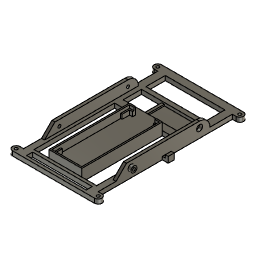
Car v2 (Autodesk Fusion 360 design; units mm, degrees)
Autodesk Fusion 360 part; units mm, degrees
note: some values were not read from the file. Set by a fixed rule: which sketch regions a step uses.
sketch "Structure" plane through (0, 0, 0) normal (0, 0, 1) x (1, 0, 0)
  line L0 (5, 0) -> (55, 0)
  line L1 (4.9996, 5) -> (5, 5)
  line L2 (5, 5) -> (5, 48)
  line L3 (4.9976, 100) -> (55, 100)
  arc A0 (55, 100) -> (54.9973, 100) centre (55, 97.5) ccw
  arc A1 (5.0024, 100) -> (4.9976, 100) centre (5, 97.5) ccw
  line L4 (10, 95) -> (10, 82)
  line L5 (10, 95) -> (50, 95)
  line L6 (50, 95) -> (50, 82)
  line L7 (10, 82) -> (50, 82)
  line L8 (10, 79) -> (10, 66.8)
  line L9 (23.6, 79) -> (10, 79)
  line L10 (10, 66.8) -> (23.6, 66.8)
  line L11 (23.6, 79) -> (23.6, 66.8)
  line L12 (4.9996, 8) -> (5, 8)
  line L13 (55, 5) -> (55, 8)
  line L14 (4.9996, 8) -> (5, 8)
  line L15 (10, 6) -> (50, 6)
  line L16 (10, 6) -> (10, 2)
  line L17 (10, 2) -> (50, 2)
  line L18 (50, 6) -> (50, 2)
  line L19 (19, 62) -> (19, 37)
  line L20 (19, 33) -> (19, 8)
  line L21 (19, 62) -> (9, 62)
  line L22 (19, 8) -> (9, 8)
  line L23 (9, 62) -> (9, 37)
  line L24 (9, 33) -> (9, 8)
  line L25 (41, 62) -> (41, 37)
  line L26 (41, 8) -> (41, 33)
  line L27 (41, 62) -> (51, 62)
  line L28 (41, 8) -> (51, 8)
  line L29 (51, 62) -> (51, 37)
  line L30 (51, 33) -> (51, 8)
  line L31 (55, 5) -> (55, 48)
  line L32 (55, 52) -> (59, 52)
  line L33 (55, 48) -> (59, 48)
  line L34 (59, 52) -> (59, 48)
  line L35 (55, 52) -> (55, 95)
  line L36 (5, 95) -> (5, 52)
  line L37 (5, 52) -> (1, 52)
  line L38 (1, 52) -> (1, 48)
  line L39 (1, 48) -> (5, 48)
  line L40 (9, 37) -> (9, 33)
  line L41 (19, 37) -> (19, 33)
  line L42 (41, 37) -> (41, 33)
  line L43 (51, 37) -> (51, 33)
  line L44 (55, 5) -> (57.5, 5)
  line L45 (55, 0) -> (57.5, 0)
  arc A2 (57.5, 0) -> (57.5, 5) centre (57.5, 2.5) ccw
  line L46 (55, 100) -> (57.5, 100)
  line L47 (55, 95) -> (57.5, 95)
  arc A3 (57.5, 95) -> (57.5, 100) centre (57.5, 97.5) ccw
  line L48 (5, 95) -> (2.5, 95)
  line L49 (5.0024, 100) -> (2.5024, 100)
  arc A4 (2.5024, 100) -> (2.5053, 95) centre (2.5, 97.5) ccw
  line L50 (4.9996, 5) -> (2.4996, 5)
  line L51 (5, 0) -> (2.5, 0)
  arc A5 (2.5006, 5) -> (2.5, 0) centre (2.5, 2.5) ccw
  dimension "d4" = 90
  dimension "d7" = 90
  dimension "d13" = 5
  dimension "d14" = 5
  dimension "d17" = 5
  dimension "d18" = 13
  dimension "d19" = 40
  dimension "d20" = 13
  dimension "d21" = 40
  dimension "d22" = 3
  dimension "d23" = 12.2
  dimension "d28" = 13.6
  dimension "d29" = 13.6
  dimension "d30" = 12.2
  dimension "d31" = 3
  dimension "d33" = 3
  dimension "d42" = 54
  dimension "d43" = 54
  dimension "d47" = 40
  dimension "d48" = 4
  dimension "d49" = 40
  dimension "d50" = 4
  dimension "d51" = 25
  dimension "d53" = 4
  dimension "d55" = 10
  dimension "d57" = 10
  dimension "d58" = 10
  dimension "d59" = 25
  dimension "d60" = 25
  dimension "d61" = 25
  dimension "d62" = 25
  dimension "d63" = 10
  dimension "d65" = 10
  dimension "d66" = 10
  dimension "d67" = 25
  dimension "d68" = 25
  dimension "d82" = 43
  dimension "d83" = 43
  dimension "d84" = 4
  dimension "d85" = 4
  dimension "d86" = 43
  dimension "d87" = 4
  dimension "d88" = 4
  dimension "d89" = 4
  dimension "d239" = 2.5
  dimension "d240" = 2.5
  dimension "d241" = 2.5
  dimension "d242" = 2.5
  dimension "d243" = 5
  dimension "d244" = 2.5
  dimension "d245" = 2.5
  dimension "d246" = 2.5
  dimension "d247" = 2.5
  constraint horizontal L0
  constraint perpendicular L1 L2
  constraint coincident L3 A0.end
  constraint coincident L3 A1.start
  constraint perpendicular L5 L6
  constraint perpendicular L6 L7
  constraint perpendicular L8 L9
  constraint perpendicular L8 L10
  constraint perpendicular L10 L11
  constraint perpendicular L2 L14
  constraint coincident L2 L12.end
  constraint perpendicular L15 L16
  constraint perpendicular L16 L17
  constraint perpendicular L15 L18
  constraint perpendicular L19 L21
  constraint perpendicular L20 L22
  constraint perpendicular L21 L23
  constraint perpendicular L25 L27
  constraint perpendicular L26 L28
  constraint perpendicular L27 L29
  constraint perpendicular L31 L33
  constraint parallel L2 L36
  constraint perpendicular L36 L37
  constraint perpendicular L37 L38
  constraint perpendicular L38 L39
  constraint parallel L24 L40
  constraint parallel L20 L41
  constraint parallel L26 L42
  constraint parallel L30 L43
  constraint perpendicular L31 L44
  constraint parallel L0 L45
  constraint parallel L3 L46
  constraint perpendicular L35 L47
  constraint perpendicular L36 L48
  constraint parallel L3 L49
  constraint coincident L48 A4.end
  constraint perpendicular L2 L50
  constraint parallel L0 L51
  constraint coincident L50 A5.start
  measures "d4" distance of L13.start L35.end
  measures "d7" distance of L1.end L36.start
  measures "d13" diameter of A0
  measures "d14" diameter of A1
  measures "d17" distance of L36.start L4.start
  measures "d18" distance of L4.start L4.end
  measures "d19" distance of L4.start L5.end
  measures "d20" distance of L5.end L6.end
  measures "d21" distance of L4.end L6.end
  measures "d22" distance of L4.end L8.start
  measures "d23" distance of L8.start L8.end
  measures "d28" distance of L9.start L8.start
  measures "d29" distance of L8.end L10.end
  measures "d30" distance of L9.start L10.end
  measures "d31" distance of L1.start L12.start
  measures "d33" distance of L13.start L13.end
  measures "d42" distance of L19.start L20.end
  measures "d43" distance of L26.start L25.start
  measures "d47" distance of L15.start L15.end
  measures "d48" distance of L15.start L16.end
  measures "d49" distance of L16.end L17.end
  measures "d50" distance of L15.end L17.end
  measures "d51" distance of L19.start L19.end
  measures "d53" distance of L19.end L20.start
  measures "d55" distance of L19.start L21.end
  measures "d57" distance of L20.start L24.start
  measures "d58" distance of L20.end L22.end
  measures "d59" distance of L21.end L23.end
  measures "d60" distance of L24.start L22.end
  measures "d61" distance of L25.start L25.end
  measures "d62" distance of L26.start L26.end
  measures "d63" distance of L25.start L27.end
  measures "d65" distance of L26.end L30.start
  measures "d66" distance of L26.start L28.end
  measures "d67" distance of L27.end L29.end
  measures "d68" distance of L30.start L28.end
  measures "d82" distance of L35.end L32.start
  measures "d83" distance of L13.start L31.end
  measures "d84" distance of L32.start L32.end
  measures "d85" distance of L31.end L33.end
  measures "d86" distance of L36.start L36.end
  measures "d87" distance of L36.end L37.end
  measures "d88" distance of L37.end L38.end
  measures "d89" distance of L38.end L2.end
  measures "d239" distance of L13.start L44.end
  measures "d240" distance of L0.end L45.end
  measures "d241" distance of L3.end L46.end
  measures "d242" distance of L35.end L47.end
  measures "d243" diameter of A3
  measures "d244" distance of L36.start L48.end
  measures "d245" distance of A1.start L49.end
  measures "d246" distance of L1.start L50.end
  measures "d247" distance of L0.start L51.end
extrude "Extrude1" add sketch "Structure" along normal blind 3
sketch "Motor Hole" plane through (0, 0, 3) normal (0, 0, 1) x (-1, 0, 0)
  line L0 (-10, -82) -> (-10, -95)
  line L1 (-10, -95) -> (-50, -95)
  line L2 (-50, -95) -> (-50, -82)
  line L3 (-50, -82) -> (-10, -82)
  line L4 (-9, -62) -> (-19, -62)
  line L5 (-19, -62) -> (-19, -8)
  line L6 (-9, -8) -> (-9, -62)
  line L7 (-10, -2) -> (-10, -6)
  line L8 (-10, -6) -> (-50, -6)
  line L9 (-50, -6) -> (-50, -2)
  line L10 (-50, -2) -> (-10, -2)
  line L11 (-10, -66.8) -> (-10, -79)
  line L12 (-10, -79) -> (-23.6, -79)
  line L13 (-23.6, -79) -> (-23.6, -66.8)
  line L14 (-23.6, -66.8) -> (-10, -66.8)
  line L15 (-41, -8) -> (-41, -62)
  line L16 (-41, -62) -> (-51, -62)
  line L17 (-51, -62) -> (-51, -8)
  line L18 (-19, -8) -> (-9, -8)
  line L19 (-51, -8) -> (-41, -8)
  line L20 (-2.5, 0) -> (-57.5, 0)
  line L21 (-55, -5) -> (-55, -48)
  arc A0 (-55, -100) -> (-54.9973, -100) centre (-55, -97.5) ccw
  line L22 (-5, -48) -> (-5, -5)
  line L23 (-50, -79) -> (-50, -66.8)
  line L24 (-50, -79) -> (-25.6, -79)
  line L25 (-25.6, -79) -> (-25.6, -66.8)
  line L26 (-25.6, -66.8) -> (-50, -66.8)
  line L27 (-23.6, -79) -> (-25.6, -79)
  line L28 (-23.6, -66.8) -> (-25.6, -66.8)
  line L29 (-5, -95) -> (-5, -52)
  line L30 (-5, -52) -> (-1, -52)
  line L31 (-1, -52) -> (-1, -48)
  line L32 (-1, -48) -> (-5, -48)
  line L33 (-55, -48) -> (-59, -48)
  line L34 (-59, -48) -> (-59, -52)
  line L35 (-59, -52) -> (-55, -52)
  line L36 (-55, -52) -> (-55, -95)
  line L37 (-5, -5) -> (-2.5006, -5)
  arc A1 (-2.5006, -5) -> (-2.5, 0) centre (-2.5, -2.5) ccw
  arc A2 (-57.5, 0) -> (-57.5, -5) centre (-57.5, -2.5) ccw
  line L38 (-57.5, -5) -> (-55, -5)
  line L39 (-55, -95) -> (-57.5, -95)
  arc A3 (-57.5, -95) -> (-57.5, -100) centre (-57.5, -97.5) ccw
  line L40 (-57.5, -100) -> (-55, -100)
  line L41 (-54.9973, -100) -> (-2.5024, -100)
  arc A4 (-2.5024, -100) -> (-2.5053, -95) centre (-2.5, -97.5) ccw
  line L42 (-2.5053, -95) -> (-5, -95)
  dimension "d71" = 3
  dimension "d72" = 12.2
  dimension "d73" = 24.4
  dimension "d74" = 12.2
  dimension "d75" = 24.4
  dimension "d76" = 2
  dimension "d77" = 2
  constraint perpendicular L3 L23
  constraint perpendicular L23 L24
  constraint perpendicular L24 L25
  constraint perpendicular L25 L26
  constraint coincident L12.end L13.start
  constraint perpendicular L25 L27
  constraint coincident L13.end L14.start
  constraint perpendicular L25 L28
  measures "d71" distance of L2.end L23.start
  measures "d72" distance of L23.start L23.end
  measures "d73" distance of L23.start L24.end
  measures "d74" distance of L24.end L25.end
  measures "d75" distance of L25.end L23.end
  measures "d76" distance of L12.end L24.end
  measures "d77" distance of L13.end L25.end
extrude "Extrude2" cut sketch "Motor Hole" against normal blind 2 contours L23 L24 L25 L26
extrude "Extrude3" cut sketch "Motor Hole" against normal blind 1 contours L13 L25 L27 L28
sketch "Rec. Base1" plane through (0, 0, 3) normal (0, 0, 1) x (-1, 0, 0)
  line L0 (-2.5, 0) -> (-57.5, 0)
  line L1 (-55, -5) -> (-55, -48)
  arc A0 (-55, -100) -> (-54.9973, -100) centre (-55, -97.5) ccw
  line L2 (-5, -48) -> (-5, -5)
  line L3 (-51, -8) -> (-41, -8)
  line L4 (-19, -8) -> (-9, -8)
  line L5 (-41, -8) -> (-41, -62)
  line L6 (-41, -62) -> (-51, -62)
  line L7 (-51, -62) -> (-51, -8)
  line L8 (-50, -66.8) -> (-10, -66.8)
  line L9 (-10, -66.8) -> (-10, -79)
  line L10 (-10, -79) -> (-50, -79)
  line L11 (-50, -79) -> (-50, -66.8)
  line L12 (-10, -2) -> (-10, -6)
  line L13 (-10, -6) -> (-50, -6)
  line L14 (-50, -6) -> (-50, -2)
  line L15 (-50, -2) -> (-10, -2)
  line L16 (-9, -62) -> (-19, -62)
  line L17 (-19, -62) -> (-19, -8)
  line L18 (-9, -8) -> (-9, -62)
  line L19 (-10, -82) -> (-10, -95)
  line L20 (-10, -95) -> (-50, -95)
  line L21 (-50, -95) -> (-50, -82)
  line L22 (-50, -82) -> (-10, -82)
  line L23 (-5, -95) -> (-5, -52)
  line L24 (-5, -52) -> (-1, -52)
  line L25 (-1, -52) -> (-1, -48)
  line L26 (-1, -48) -> (-5, -48)
  line L27 (-55, -48) -> (-59, -48)
  line L28 (-59, -48) -> (-59, -52)
  line L29 (-59, -52) -> (-55, -52)
  line L30 (-55, -52) -> (-55, -95)
  line L31 (-19, -8) -> (-41, -8)
  line L32 (-19, -8) -> (-19, -62)
  line L33 (-41, -8) -> (-41, -62)
  line L34 (-19, -62) -> (-26, -62)
  line L35 (-41, -62) -> (-34, -62)
  line L36 (-26, -62) -> (-26, -61)
  line L37 (-34, -62) -> (-34, -61)
  line L38 (-26, -61) -> (-20, -61)
  line L39 (-34, -61) -> (-40, -61)
  line L40 (-20, -61) -> (-20, -9)
  line L41 (-20, -9) -> (-40, -9)
  line L42 (-40, -9) -> (-40, -61)
  line L43 (-5, -5) -> (-2.5006, -5)
  arc A1 (-2.5006, -5) -> (-2.5, 0) centre (-2.5, -2.5) ccw
  arc A2 (-57.5, 0) -> (-57.5, -5) centre (-57.5, -2.5) ccw
  line L44 (-57.5, -5) -> (-55, -5)
  line L45 (-55, -95) -> (-57.5, -95)
  arc A3 (-57.5, -95) -> (-57.5, -100) centre (-57.5, -97.5) ccw
  line L46 (-57.5, -100) -> (-55, -100)
  line L47 (-54.9973, -100) -> (-2.5024, -100)
  arc A4 (-2.5024, -100) -> (-2.5053, -95) centre (-2.5, -97.5) ccw
  line L48 (-2.5053, -95) -> (-5, -95)
  dimension "d90" = 22
  dimension "d91" = 54
  dimension "d92" = 54
  dimension "d93" = 7
  dimension "d94" = 7
  dimension "d95" = 1
  dimension "d96" = 1
  dimension "d97" = 6
  dimension "d98" = 6
  dimension "d99" = 52
  dimension "d100" = 20
  dimension "d101" = 52
  constraint coincident L4.start L17.end
  constraint perpendicular L16 L32
  constraint perpendicular L6 L33
  constraint coincident L16.end L17.start
  constraint perpendicular L32 L34
  constraint coincident L5.end L6.start
  constraint perpendicular L33 L35
  constraint perpendicular L34 L36
  constraint perpendicular L35 L37
  constraint perpendicular L36 L38
  constraint perpendicular L37 L39
  constraint perpendicular L38 L40
  constraint perpendicular L32 L41
  constraint perpendicular L41 L42
  measures "d90" distance of L4.start L3.end
  measures "d91" distance of L4.start L16.end
  measures "d92" distance of L3.end L5.end
  measures "d93" distance of L16.end L34.end
  measures "d94" distance of L5.end L35.end
  measures "d95" distance of L34.end L36.end
  measures "d96" distance of L35.end L37.end
  measures "d97" distance of L36.end L38.end
  measures "d98" distance of L37.end L39.end
  measures "d99" distance of L38.end L40.end
  measures "d100" distance of L40.end L41.end
  measures "d101" distance of L41.end L39.end
extrude "Extrude4" add sketch "Rec. Base1" along normal blind 7 contours L5 L17 L31 L32 L33 L34 L35 L36 L37 L38 L39 L40 L41 L42
sketch "Hook" plane through (0, 0, 3) normal (0, 0, 1) x (-1, 0, 0)
  line L0 (-34, -62) -> (-41, -62)
  line L1 (-41, -62) -> (-51, -62)
  line L2 (-51, -62) -> (-51, -8)
  line L3 (-51, -8) -> (-41, -8)
  line L4 (-41, -8) -> (-19, -8)
  line L5 (-19, -8) -> (-9, -8)
  line L6 (-9, -8) -> (-9, -62)
  line L7 (-9, -62) -> (-19, -62)
  line L8 (-19, -62) -> (-26, -62)
  line L9 (-26, -62) -> (-26, -61)
  line L10 (-26, -61) -> (-20, -61)
  line L11 (-20, -61) -> (-20, -9)
  line L12 (-20, -9) -> (-40, -9)
  line L13 (-40, -9) -> (-40, -61)
  line L14 (-40, -61) -> (-34, -61)
  line L15 (-34, -61) -> (-34, -62)
  arc A0 (-55, -100) -> (-54.9973, -100) centre (-55, -97.5) ccw
  line L16 (-5, -95) -> (-5, -52)
  line L17 (-5, -52) -> (-1, -52)
  line L18 (-1, -52) -> (-1, -48)
  line L19 (-1, -48) -> (-5, -48)
  line L20 (-5, -48) -> (-5, -5)
  line L21 (-2.5, 0) -> (-57.5, 0)
  line L22 (-55, -5) -> (-55, -48)
  line L23 (-55, -48) -> (-59, -48)
  line L24 (-59, -48) -> (-59, -52)
  line L25 (-59, -52) -> (-55, -52)
  line L26 (-55, -52) -> (-55, -95)
  line L27 (-10, -2) -> (-10, -6)
  line L28 (-10, -6) -> (-50, -6)
  line L29 (-50, -6) -> (-50, -2)
  line L30 (-50, -2) -> (-10, -2)
  line L31 (-50, -66.8) -> (-10, -66.8)
  line L32 (-10, -66.8) -> (-10, -79)
  line L33 (-10, -79) -> (-50, -79)
  line L34 (-50, -79) -> (-50, -66.8)
  line L35 (-10, -82) -> (-10, -95)
  line L36 (-10, -95) -> (-50, -95)
  line L37 (-50, -95) -> (-50, -82)
  line L38 (-50, -82) -> (-10, -82)
  line L39 (-57, -52) -> (-57, -48)
  line L40 (-55, -52) -> (-55, -48)
  line L41 (-5, -52) -> (-5, -48)
  line L42 (-3, -52) -> (-3, -48)
  line L43 (-5, -5) -> (-2.5006, -5)
  arc A1 (-2.5006, -5) -> (-2.5, 0) centre (-2.5, -2.5) ccw
  arc A2 (-57.5, 0) -> (-57.5, -5) centre (-57.5, -2.5) ccw
  line L44 (-57.5, -5) -> (-55, -5)
  line L45 (-55, -95) -> (-57.5, -95)
  arc A3 (-57.5, -95) -> (-57.5, -100) centre (-57.5, -97.5) ccw
  line L46 (-57.5, -100) -> (-55, -100)
  line L47 (-54.9973, -100) -> (-2.5024, -100)
  arc A4 (-2.5024, -100) -> (-2.5053, -95) centre (-2.5, -97.5) ccw
  line L48 (-2.5053, -95) -> (-5, -95)
  constraint midpoint L25 L39.start
  constraint midpoint L23 L39.end
  constraint coincident L25.end L26.start
  constraint coincident L22.end L23.start
  constraint coincident L16.end L17.start
  constraint coincident L19.end L20.start
  constraint midpoint L17 L42.start
  constraint midpoint L19 L42.end
extrude "Extrude5" cut sketch "Hook" against normal blind 1 contours L23 L25 L39 L40
extrude "Extrude6" add 1 faces at (57.6667, 50.6667, 3) along direction (0, 0, 1) blind 1
extrude "Extrude7" cut sketch "Hook" against normal blind 1 contours L17 L19 L41 L42
extrude "Extrude8" add sketch "Hook" along normal blind 1 contours L17 L18 L19 L42
sketch "Rec. Base2" plane through (0, 0, 3) normal (0, 0, 1) x (-1, 0, 0)
  line L0 (-5, -95) -> (-5, -5)
  line L1 (-2.5, 0) -> (-57.5, 0)
  line L2 (-55, -5) -> (-55, -95)
  arc A0 (-55, -100) -> (-54.9973, -100) centre (-55, -97.5) ccw
  line L3 (-34, -62) -> (-41, -62)
  line L4 (-41, -62) -> (-51, -62)
  line L5 (-51, -62) -> (-51, -8)
  line L6 (-51, -8) -> (-41, -8)
  line L7 (-41, -8) -> (-19, -8)
  line L8 (-19, -8) -> (-9, -8)
  line L9 (-9, -8) -> (-9, -62)
  line L10 (-9, -62) -> (-19, -62)
  line L11 (-19, -62) -> (-26, -62)
  line L12 (-26, -62) -> (-26, -61)
  line L13 (-26, -61) -> (-20, -61)
  line L14 (-20, -61) -> (-20, -9)
  line L15 (-20, -9) -> (-40, -9)
  line L16 (-40, -9) -> (-40, -61)
  line L17 (-40, -61) -> (-34, -61)
  line L18 (-34, -61) -> (-34, -62)
  line L19 (-10, -2) -> (-10, -6)
  line L20 (-10, -6) -> (-50, -6)
  line L21 (-50, -6) -> (-50, -2)
  line L22 (-50, -2) -> (-10, -2)
  line L23 (-50, -66.8) -> (-10, -66.8)
  line L24 (-10, -66.8) -> (-10, -79)
  line L25 (-10, -79) -> (-50, -79)
  line L26 (-50, -79) -> (-50, -66.8)
  line L27 (-10, -82) -> (-10, -95)
  line L28 (-10, -95) -> (-50, -95)
  line L29 (-50, -95) -> (-50, -82)
  line L30 (-50, -82) -> (-10, -82)
  line L31 (-20, -58) -> (-21, -58)
  line L32 (-21, -58) -> (-21, -60)
  line L33 (-21, -60) -> (-23, -60)
  line L34 (-23, -60) -> (-23, -61)
  line L35 (-40, -58) -> (-39, -58)
  line L36 (-39, -58) -> (-39, -60)
  line L37 (-39, -60) -> (-37, -60)
  line L38 (-37, -60) -> (-37, -61)
  line L39 (-20, -12) -> (-21, -12)
  line L40 (-21, -12) -> (-21, -10)
  line L41 (-21, -10) -> (-23, -10)
  line L42 (-23, -10) -> (-23, -9)
  line L43 (-40, -12) -> (-39, -12)
  line L44 (-39, -12) -> (-39, -10)
  line L45 (-39, -10) -> (-37, -10)
  line L46 (-37, -10) -> (-37, -9)
  line L47 (-5, -5) -> (-2.5006, -5)
  arc A1 (-2.5006, -5) -> (-2.5, 0) centre (-2.5, -2.5) ccw
  arc A2 (-57.5, 0) -> (-57.5, -5) centre (-57.5, -2.5) ccw
  line L48 (-57.5, -5) -> (-55, -5)
  line L49 (-55, -95) -> (-57.5, -95)
  arc A3 (-57.5, -95) -> (-57.5, -100) centre (-57.5, -97.5) ccw
  line L50 (-57.5, -100) -> (-55, -100)
  line L51 (-54.9973, -100) -> (-2.5024, -100)
  arc A4 (-2.5024, -100) -> (-2.5053, -95) centre (-2.5, -97.5) ccw
  line L52 (-2.5053, -95) -> (-5, -95)
  dimension "d112" = 3
  dimension "d113" = 1
  dimension "d114" = 2
  dimension "d115" = 2
  dimension "d116" = 1
  dimension "d117" = 3
  dimension "d118" = 1
  dimension "d119" = 2
  dimension "d120" = 2
  dimension "d121" = 1
  dimension "d122" = 3
  dimension "d123" = 1
  dimension "d124" = 2
  dimension "d125" = 2
  dimension "d126" = 1
  dimension "d127" = 3
  dimension "d128" = 1
  dimension "d129" = 2
  dimension "d130" = 2
  dimension "d131" = 1
  constraint perpendicular L31 L32
  constraint perpendicular L32 L33
  constraint perpendicular L13 L34
  constraint perpendicular L35 L36
  constraint perpendicular L36 L37
  constraint perpendicular L37 L38
  constraint perpendicular L39 L40
  constraint perpendicular L40 L41
  constraint perpendicular L41 L42
  constraint perpendicular L43 L44
  constraint perpendicular L44 L45
  constraint perpendicular L45 L46
  measures "d112" distance of L13.end L31.start
  measures "d113" distance of L31.start L31.end
  measures "d114" distance of L31.end L32.end
  measures "d115" distance of L32.end L33.end
  measures "d116" distance of L33.end L34.end
  measures "d117" distance of L16.end L35.start
  measures "d118" distance of L35.start L35.end
  measures "d119" distance of L35.end L36.end
  measures "d120" distance of L36.end L37.end
  measures "d121" distance of L37.end L38.end
  measures "d122" distance of L14.end L39.start
  measures "d123" distance of L39.start L39.end
  measures "d124" distance of L39.end L40.end
  measures "d125" distance of L40.end L41.end
  measures "d126" distance of L41.end L42.end
  measures "d127" distance of L15.end L43.start
  measures "d128" distance of L43.start L43.end
  measures "d129" distance of L43.end L44.end
  measures "d130" distance of L44.end L45.end
  measures "d131" distance of L45.end L46.end
extrude "Extrude9" cut 1 faces at (40.6667, 26.3333, 10) along direction (0, 0, -1) blind 2
extrude "Extrude10" add sketch "Rec. Base2" along normal blind 3 contours L13 L14 L31 L32 L33 L34
extrude "Extrude11" add sketch "Rec. Base2" along normal blind 3 contours L16 L17 L35 L36 L37 L38
extrude "Extrude12" add sketch "Rec. Base2" along normal blind 3 contours L15 L16 L43 L44 L45 L46
extrude "Extrude13" add sketch "Rec. Base2" along normal blind 3 contours L14 L15 L39 L40 L41 L42
sketch "Side Wheel Base" plane through (0, 0, 3) normal (0, 0, 1) x (-1, 0, 0)
  line L0 (-5, -95) -> (-5, -5)
  line L1 (-2.5, 0) -> (-57.5, 0)
  line L2 (-55, -5) -> (-55, -95)
  arc A0 (-55, -100) -> (-54.9973, -100) centre (-55, -97.5) ccw
  line L3 (-10, -2) -> (-10, -6)
  line L4 (-10, -6) -> (-50, -6)
  line L5 (-50, -6) -> (-50, -2)
  line L6 (-50, -2) -> (-10, -2)
  line L7 (-50, -66.8) -> (-10, -66.8)
  line L8 (-10, -66.8) -> (-10, -79)
  line L9 (-10, -79) -> (-50, -79)
  line L10 (-50, -79) -> (-50, -66.8)
  line L11 (-10, -82) -> (-10, -95)
  line L12 (-10, -95) -> (-50, -95)
  line L13 (-50, -95) -> (-50, -82)
  line L14 (-50, -82) -> (-10, -82)
  line L15 (-20, -12) -> (-21, -12)
  line L16 (-21, -12) -> (-21, -10)
  line L17 (-21, -10) -> (-23, -10)
  line L18 (-23, -10) -> (-23, -9)
  line L19 (-23, -9) -> (-37, -9)
  line L20 (-37, -9) -> (-37, -10)
  line L21 (-37, -10) -> (-39, -10)
  line L22 (-39, -10) -> (-39, -12)
  line L23 (-39, -12) -> (-40, -12)
  line L24 (-40, -12) -> (-40, -58)
  line L25 (-40, -58) -> (-39, -58)
  line L26 (-39, -58) -> (-39, -60)
  line L27 (-39, -60) -> (-37, -60)
  line L28 (-37, -60) -> (-37, -61)
  line L29 (-37, -61) -> (-34, -61)
  line L30 (-34, -61) -> (-34, -62)
  line L31 (-34, -62) -> (-41, -62)
  line L32 (-41, -62) -> (-51, -62)
  line L33 (-51, -62) -> (-51, -8)
  line L34 (-51, -8) -> (-41, -8)
  line L35 (-41, -8) -> (-19, -8)
  line L36 (-19, -8) -> (-9, -8)
  line L37 (-9, -8) -> (-9, -62)
  line L38 (-9, -62) -> (-19, -62)
  line L39 (-19, -62) -> (-26, -62)
  line L40 (-26, -62) -> (-26, -61)
  line L41 (-26, -61) -> (-23, -61)
  line L42 (-23, -61) -> (-23, -60)
  line L43 (-23, -60) -> (-21, -60)
  line L44 (-21, -60) -> (-21, -58)
  line L45 (-21, -58) -> (-20, -58)
  line L46 (-20, -58) -> (-20, -12)
  circle A1 centre (-5, -2.5) radius 1.5
  circle A2 centre (-55, -2.5) radius 1.5
  circle A3 centre (-55, -97.5) radius 1.5
  circle A4 centre (-5, -97.5) radius 1.5
  circle A5 centre (-5, -97.5) radius 0.9
  circle A6 centre (-55, -97.5) radius 0.9
  circle A7 centre (-55, -2.5) radius 0.9
  circle A8 centre (-5, -2.5) radius 0.9
  line L47 (-5, -5) -> (-2.5006, -5)
  arc A9 (-2.5006, -5) -> (-2.5, 0) centre (-2.5, -2.5) ccw
  arc A10 (-57.5, 0) -> (-57.5, -5) centre (-57.5, -2.5) ccw
  line L48 (-57.5, -5) -> (-55, -5)
  line L49 (-55, -95) -> (-57.5, -95)
  arc A11 (-57.5, -95) -> (-57.5, -100) centre (-57.5, -97.5) ccw
  line L50 (-57.5, -100) -> (-55, -100)
  line L51 (-54.9973, -100) -> (-2.5024, -100)
  arc A12 (-2.5024, -100) -> (-2.5053, -95) centre (-2.5, -97.5) ccw
  line L52 (-2.5053, -95) -> (-5, -95)
  dimension "d142" = 3
  dimension "d143" = 3
  dimension "d144" = 3
  dimension "d145" = 3
  dimension "d146" = 1.8
  dimension "d147" = 1.8
  dimension "d148" = 1.8
  dimension "d149" = 1.8
  constraint concentric A0 A3
  constraint concentric A4 A5
  constraint concentric A3 A6
  constraint concentric A2 A7
  constraint concentric A1 A8
  measures "d142" diameter of A1
  measures "d143" diameter of A2
  measures "d144" diameter of A3
  measures "d145" diameter of A4
  measures "d146" diameter of A5
  measures "d147" diameter of A6
  measures "d148" diameter of A7
  measures "d149" diameter of A8
extrude "Extrude14" add sketch "Side Wheel Base" along normal blind 3.4 contours A8
extrude "Extrude15" add sketch "Side Wheel Base" along normal blind 1 contours A1
extrude "Extrude16" add sketch "Side Wheel Base" along normal blind 3.4 contours A7
extrude "Extrude17" add sketch "Side Wheel Base" along normal blind 1 contours A2
extrude "Extrude18" add sketch "Side Wheel Base" along normal blind 3.4 contours A6
extrude "Extrude19" add sketch "Side Wheel Base" along normal blind 1 contours A3
extrude "Extrude20" add sketch "Side Wheel Base" along normal blind 3.4 contours A5
extrude "Extrude21" add sketch "Side Wheel Base" along normal blind 1 contours A4
sketch "Side Car1" plane through (0, 0, 3) normal (0, 0, 1) x (-1, 0, 0)
  circle A0 centre (-5, -97.5) radius 1.5
  circle A1 centre (-55, -97.5) radius 1.5
  circle A2 centre (-55, -2.5) radius 1.5
  circle A3 centre (-5, -2.5) radius 1.5
  line L0 (-5, -95) -> (-5, -5)
  line L1 (-2.5, 0) -> (-57.5, 0)
  line L2 (-55, -5) -> (-55, -95)
  arc A4 (-55, -100) -> (-54.9973, -100) centre (-55, -97.5) ccw
  line L3 (-10, -2) -> (-10, -6)
  line L4 (-10, -6) -> (-50, -6)
  line L5 (-50, -6) -> (-50, -2)
  line L6 (-50, -2) -> (-10, -2)
  line L7 (-50, -66.8) -> (-10, -66.8)
  line L8 (-10, -66.8) -> (-10, -79)
  line L9 (-10, -79) -> (-50, -79)
  line L10 (-50, -79) -> (-50, -66.8)
  line L11 (-10, -82) -> (-10, -95)
  line L12 (-10, -95) -> (-50, -95)
  line L13 (-50, -95) -> (-50, -82)
  line L14 (-50, -82) -> (-10, -82)
  line L15 (-20, -12) -> (-21, -12)
  line L16 (-21, -12) -> (-21, -10)
  line L17 (-21, -10) -> (-23, -10)
  line L18 (-23, -10) -> (-23, -9)
  line L19 (-23, -9) -> (-37, -9)
  line L20 (-37, -9) -> (-37, -10)
  line L21 (-37, -10) -> (-39, -10)
  line L22 (-39, -10) -> (-39, -12)
  line L23 (-39, -12) -> (-40, -12)
  line L24 (-40, -12) -> (-40, -58)
  line L25 (-40, -58) -> (-39, -58)
  line L26 (-39, -58) -> (-39, -60)
  line L27 (-39, -60) -> (-37, -60)
  line L28 (-37, -60) -> (-37, -61)
  line L29 (-37, -61) -> (-34, -61)
  line L30 (-34, -61) -> (-34, -62)
  line L31 (-34, -62) -> (-41, -62)
  line L32 (-41, -62) -> (-51, -62)
  line L33 (-51, -62) -> (-51, -8)
  line L34 (-51, -8) -> (-41, -8)
  line L35 (-41, -8) -> (-19, -8)
  line L36 (-19, -8) -> (-9, -8)
  line L37 (-9, -8) -> (-9, -62)
  line L38 (-9, -62) -> (-19, -62)
  line L39 (-19, -62) -> (-26, -62)
  line L40 (-26, -62) -> (-26, -61)
  line L41 (-26, -61) -> (-23, -61)
  line L42 (-23, -61) -> (-23, -60)
  line L43 (-23, -60) -> (-21, -60)
  line L44 (-21, -60) -> (-21, -58)
  line L45 (-21, -58) -> (-20, -58)
  line L46 (-20, -58) -> (-20, -12)
  line L47 (-55, -80) -> (-53, -80)
  line L48 (-55, -17) -> (-53, -17)
  line L49 (-53, -80) -> (-53, -17)
  line L50 (-5, -80) -> (-7, -80)
  line L51 (-7, -80) -> (-7, -17)
  line L52 (-5, -17) -> (-7, -17)
  line L53 (-5, -5) -> (-2.5006, -5)
  arc A5 (-2.5006, -5) -> (-2.5, 0) centre (-2.5, -2.5) ccw
  arc A6 (-57.5, 0) -> (-57.5, -5) centre (-57.5, -2.5) ccw
  line L54 (-57.5, -5) -> (-55, -5)
  line L55 (-55, -95) -> (-57.5, -95)
  arc A7 (-57.5, -95) -> (-57.5, -100) centre (-57.5, -97.5) ccw
  line L56 (-57.5, -100) -> (-55, -100)
  line L57 (-54.9973, -100) -> (-2.5024, -100)
  arc A8 (-2.5024, -100) -> (-2.5053, -95) centre (-2.5, -97.5) ccw
  line L58 (-2.5053, -95) -> (-5, -95)
  dimension "d166" = 12
  dimension "d167" = 15
  dimension "d168" = 2
  dimension "d169" = 2
  dimension "d170" = 63
  dimension "d171" = 15
  dimension "d172" = 12
  dimension "d173" = 2
  dimension "d174" = 63
  dimension "d175" = 2
  constraint perpendicular L48 L49
  constraint perpendicular L50 L51
  constraint perpendicular L51 L52
  measures "d166" distance of L2.start L48.start
  measures "d167" distance of L2.end L47.start
  measures "d168" distance of L47.start L47.end
  measures "d169" distance of L48.start L48.end
  measures "d170" distance of L47.end L48.end
  measures "d171" distance of L0.start L50.start
  measures "d172" distance of L0.end L52.start
  measures "d173" distance of L50.start L50.end
  measures "d174" distance of L50.end L51.end
  measures "d175" distance of L52.start L51.end
extrude "Extrude22" add sketch "Side Car1" along normal blind 7 contours L0 L50 L51 L52
extrude "Extrude23" add sketch "Side Car1" along normal blind 7 contours L2 L47 L48 L49
sketch "Left Side Car" plane through (55, 0, 0) normal (1, 0, 0) x (0, 1, 0)
  line L0 (52, 0) -> (95, 0)
  line L1 (95, 3) -> (80, 3)
  line L2 (80, 3) -> (80, 10)
  line L3 (80, 10) -> (17, 10)
  line L4 (17, 10) -> (17, 3)
  line L5 (48, 0) -> (48, 2)
  line L6 (48, 2) -> (52, 2)
  line L7 (52, 2) -> (52, 0)
  line L8 (17, 3) -> (24, 10)
  arc A0 (80, 3) -> (73, 10) centre (73, 3) ccw
  line L9 (95, 0) -> (95, 3)
  line L10 (17, 3) -> (5, 3)
  line L11 (5, 3) -> (5, 0)
  line L12 (5, 0) -> (48, 0)
  dimension "d182" = 7
  dimension "d183" = 14
  constraint coincident L4.end L8.start
  constraint coincident L3 A0.end
  measures "d182" distance of L1.end A0.centre
  measures "d183" diameter of A0
extrude "Extrude24" cut sketch "Left Side Car" against normal blind 3 contours L3 L4 L8
extrude "Extrude25" cut sketch "Left Side Car" against normal blind 3 contours L2 L3 A0
sketch "Right Side Car" plane through (5, 0, 0) normal (-1, 0, 0) x (0, -1, 0)
  line L0 (-48, 0) -> (-5, 0)
  line L1 (-5, 0) -> (-5, 3)
  line L2 (-5, 3) -> (-17, 3)
  line L3 (-17, 3) -> (-17, 10)
  line L4 (-17, 10) -> (-80, 10)
  line L5 (-80, 10) -> (-80, 3)
  line L6 (-52, 0) -> (-52, 2)
  line L7 (-52, 2) -> (-48, 2)
  line L8 (-48, 2) -> (-48, 0)
  line L9 (-24, 10) -> (-17, 3)
  arc A0 (-73, 10) -> (-80, 3) centre (-73, 3) ccw
  line L10 (-80, 3) -> (-95, 3)
  line L11 (-95, 3) -> (-95, 0)
  line L12 (-95, 0) -> (-52, 0)
  dimension "d190" = 7
  dimension "d191" = 14
  constraint coincident L2.end L3.start
  constraint coincident L4 A0.start
  measures "d190" distance of L5.end A0.centre
  measures "d191" diameter of A0
extrude "Extrude26" cut sketch "Right Side Car" against normal blind 3 contours L4 L5 A0
extrude "Extrude27" cut sketch "Right Side Car" against normal blind 3 contours L3 L4 L9
sketch "Left Base Wheel" plane through (55, 0, 0) normal (1, 0, 0) x (0, 1, 0)
  arc A0 (80, 3) -> (73, 10) centre (73, 3) ccw
  line L0 (73, 10) -> (24, 10)
  line L1 (24, 10) -> (17, 3)
  line L2 (17, 3) -> (5, 3)
  line L3 (5, 0) -> (48, 0)
  line L4 (48, 0) -> (48, 2)
  line L5 (48, 2) -> (52, 2)
  line L6 (52, 2) -> (52, 0)
  line L7 (52, 0) -> (95, 0)
  line L8 (95, 3) -> (80, 3)
  circle A1 centre (27, 6) radius 2
  circle A2 centre (27, 6) radius 1
  circle A3 centre (73, 6) radius 2
  line L9 (5, 3) -> (5, 0)
  line L10 (95, 0) -> (95, 3)
  dimension "d198" = 4
  dimension "d199" = 2
  dimension "d202" = 4
  constraint concentric A1 A2
  measures "d198" diameter of A1
  measures "d199" diameter of A2
  measures "d202" diameter of A3
extrude "Extrude28" cut sketch "Left Base Wheel" against normal blind 3 contours A3
extrude "Extrude29" add sketch "Left Base Wheel" along normal blind 4.4 contours A2
extrude "Extrude30" add sketch "Left Base Wheel" along normal blind 2 contours A1
sketch "Right Base Wheel" plane through (5, 0, 0) normal (-1, 0, 0) x (0, -1, 0)
  line L0 (-17, 3) -> (-24, 10)
  line L1 (-24, 10) -> (-73, 10)
  arc A0 (-73, 10) -> (-80, 3) centre (-73, 3) ccw
  line L2 (-80, 3) -> (-95, 3)
  line L3 (-95, 0) -> (-52, 0)
  line L4 (-52, 0) -> (-52, 2)
  line L5 (-52, 2) -> (-48, 2)
  line L6 (-48, 2) -> (-48, 0)
  line L7 (-48, 0) -> (-5, 0)
  line L8 (-5, 0) -> (-5, 3)
  line L9 (-5, 3) -> (-17, 3)
  circle A1 centre (-73, 6) radius 2
  circle A2 centre (-73, 6) radius 1
  circle A3 centre (-27, 6) radius 2
  circle A4 centre (-27, 6) radius 1
  line L10 (-95, 3) -> (-95, 0)
  dimension "d211" = 4
  dimension "d212" = 2
  dimension "d215" = 4
  dimension "d216" = 2
  constraint concentric A1 A2
  constraint concentric A3 A4
  measures "d211" diameter of A1
  measures "d212" diameter of A2
  measures "d215" diameter of A3
  measures "d216" diameter of A4
extrude "Extrude31" add sketch "Right Base Wheel" along normal blind 4.4 contours A2
extrude "Extrude32" add sketch "Right Base Wheel" along normal blind 2 contours A1
extrude "Extrude33" add sketch "Right Base Wheel" along normal blind 4.4 contours A4
extrude "Extrude34" add sketch "Right Base Wheel" along normal blind 2 contours A3
extrude "Extrude35" add 1 faces at (20.3333, 12, 4) along direction (0, 1, 0) blind 3
extrude "Extrude36" add 1 faces at (20.3333, 58, 4) along direction (0, -1, 0) blind 3
extrude "Extrude37" add 1 faces at (39.6667, 58, 4) along direction (0, -1, 0) blind 3
extrude "Extrude38" add 1 faces at (39.6667, 12, 4) along direction (0, 1, 0) blind 3
extrude "Extrude39" cut 1 faces at (25.6, 74.9333, 1.6667) along direction (-1, 0, 0) blind 0.2
extrude "Extrude40" cut 1 faces at (26, 61.6667, 4.6667) along direction (-1, 0, 0) blind 3
extrude "Extrude41" cut 1 faces at (34, 61.6667, 4.6667) along direction (1, 0, 0) blind 3
extrude "Extrude42" cut 1 faces at (56.2589, 97.8103, 4) along direction (0, 0, -1) blind 1
extrude "Extrude43" cut 1 faces at (55.0668, 97.2075, 6.4) along direction (0, 0, -1) blind 3.4
extrude "Extrude44" cut 1 faces at (6.1986, 97.0055, 4) along direction (0, 0, -1) blind 1
extrude "Extrude45" cut 1 faces at (5.4671, 97.669, 6.4) along direction (0, 0, -1) blind 3.4
extrude "Extrude46" cut 1 faces at (53.7089, 2.6192, 4) along direction (0, 0, -1) blind 1
extrude "Extrude47" cut 1 faces at (54.3598, 2.6859, 6.4) along direction (0, 0, -1) blind 3.4
extrude "Extrude48" cut 1 faces at (3.7089, 2.6192, 4) along direction (0, 0, -1) blind 1
extrude "Extrude49" cut 1 faces at (4.603, 2.6636, 6.4) along direction (0, 0, -1) blind 3.4
sketch "Sketch13" plane through (0, 0, 3) normal (0, 0, 1) x (-1, 0, 0)
  line L0 (-39, -15) -> (-40, -15)
  line L1 (-40, -15) -> (-40, -55)
  line L2 (-40, -55) -> (-39, -55)
  line L3 (-39, -55) -> (-39, -60)
  line L4 (-39, -60) -> (-37, -60)
  line L5 (-37, -60) -> (-37, -62)
  line L6 (-37, -62) -> (-41, -62)
  line L7 (-41, -62) -> (-51, -62)
  line L8 (-51, -62) -> (-51, -8)
  line L9 (-51, -8) -> (-41, -8)
  line L10 (-41, -8) -> (-19, -8)
  line L11 (-19, -8) -> (-9, -8)
  line L12 (-9, -8) -> (-9, -62)
  line L13 (-9, -62) -> (-19, -62)
  line L14 (-19, -62) -> (-23, -62)
  line L15 (-23, -62) -> (-23, -60)
  line L16 (-23, -60) -> (-21, -60)
  line L17 (-21, -60) -> (-21, -55)
  line L18 (-21, -55) -> (-20, -55)
  line L19 (-20, -55) -> (-20, -15)
  line L20 (-20, -15) -> (-21, -15)
  line L21 (-21, -15) -> (-21, -10)
  line L22 (-21, -10) -> (-23, -10)
  line L23 (-23, -10) -> (-23, -9)
  line L24 (-23, -9) -> (-37, -9)
  line L25 (-37, -9) -> (-37, -10)
  line L26 (-37, -10) -> (-39, -10)
  line L27 (-39, -10) -> (-39, -15)
  line L28 (-10, -2) -> (-10, -6)
  line L29 (-10, -6) -> (-50, -6)
  line L30 (-50, -6) -> (-50, -2)
  line L31 (-50, -2) -> (-10, -2)
  line L32 (-10, -82) -> (-10, -95)
  line L33 (-10, -95) -> (-50, -95)
  line L34 (-50, -95) -> (-50, -82)
  line L35 (-50, -82) -> (-10, -82)
  line L36 (-50, -66.8) -> (-10, -66.8)
  line L37 (-10, -66.8) -> (-10, -79)
  line L38 (-10, -79) -> (-50, -79)
  line L39 (-50, -79) -> (-50, -66.8)
  line L40 (-53, -80) -> (-55, -80)
  line L41 (-55, -80) -> (-55, -95)
  line L42 (-55, -95) -> (-57.5, -95)
  arc A0 (-57.5, -95) -> (-57.5, -100) centre (-57.5, -97.5) ccw
  line L43 (-57.5, -100) -> (-55, -100)
  arc A1 (-55, -100) -> (-54.9973, -100) centre (-55, -97.5) ccw
  line L44 (-54.9973, -100) -> (-2.5024, -100)
  arc A2 (-2.5024, -100) -> (-2.5053, -95) centre (-2.5, -97.5) ccw
  line L45 (-2.5053, -95) -> (-5, -95)
  line L46 (-5, -95) -> (-5, -80)
  line L47 (-5, -80) -> (-7, -80)
  line L48 (-7, -80) -> (-7, -17)
  line L49 (-7, -17) -> (-5, -17)
  line L50 (-5, -17) -> (-5, -5)
  line L51 (-5, -5) -> (-2.5006, -5)
  arc A3 (-2.5006, -5) -> (-2.5, 0) centre (-2.5, -2.5) ccw
  line L52 (-2.5, 0) -> (-57.5, 0)
  arc A4 (-57.5, 0) -> (-57.5, -5) centre (-57.5, -2.5) ccw
  line L53 (-57.5, -5) -> (-55, -5)
  line L54 (-55, -5) -> (-55, -17)
  line L55 (-55, -17) -> (-53, -17)
  line L56 (-53, -17) -> (-53, -80)
  circle A5 centre (-2.5, -2.5) radius 1
  circle A6 centre (-57.5, -2.5) radius 1
  circle A7 centre (-57.5, -97.5) radius 1
  circle A8 centre (-2.5, -97.5) radius 1
  dimension "d264" = 2
  dimension "d265" = 2
  dimension "d266" = 2
  dimension "d267" = 2
  constraint concentric A3 A5
  constraint concentric A4 A6
  constraint concentric A0 A7
  constraint concentric A2 A8
  measures "d264" diameter of A5
  measures "d265" diameter of A6
  measures "d266" diameter of A7
  measures "d267" diameter of A8
extrude "Extrude50" cut sketch "Sketch13" against normal blind 4 contours A6
extrude "Extrude51" cut sketch "Sketch13" against normal blind 4 contours A5
extrude "Extrude52" cut sketch "Sketch13" against normal blind 4 contours A8
extrude "Extrude53" cut sketch "Sketch13" against normal blind 4 contours A7
extrude "Extrude54" cut 1 faces at (59.4, 26.9258, 6.325) along direction (-1, 0, 0) blind 2.4
extrude "Extrude55" cut 1 faces at (0.6, 27.0742, 6.325) along direction (1, 0, 0) blind 2.4
extrude "Extrude56" cut 1 faces at (0.6, 73.0787, 5.4037) along direction (1, 0, 0) blind 2.4
extrude "Extrude57" cut sketch "Left Base Wheel" along normal blind 3 and the other way blind 3 contours A2
extrude "Extrude58" cut sketch "Right Base Wheel" along normal blind 3 and the other way blind 3 contours A2
extrude "Extrude59" cut sketch "Right Base Wheel" along normal blind 3 and the other way blind 3 contours A4
